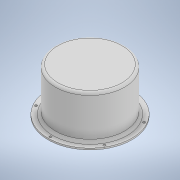
# Autodesk Inventor part: Cover_Joint_1_2
Saved by Autodesk Inventor 2021 (Build 250183000, 183)
## iProperties
Created: 2020-05-10
Part Number: Cover_Joint_1_2
Material: Generic
Document SubType Name: Modeling
Designer: avi41
Density: 1 g/cm^3
Appearance: Default
Mass: 384.639 g
Surface Area: 3507.09 cm^2
Volume: 384.639 cm^3
Author: avi41
Autodesk Inventor part; units mm, degrees
ref_plane "YZ Plane" through (0, 0, 0) normal (1, 0, 0) x (0, 1, 0)
ref_plane "XZ Plane" through (0, 0, 0) normal (0, 1, 0) x (-1, 0, 0)
ref_plane "XY Plane" through (0, 0, 0) normal (0, 0, 1) x (1, 0, 0)
sketch "Sketch1" plane through (0, 0, 0) normal (0, 0, 1) x (1, 0, 0)
  line L0 (-16.3, 0) -> (97.8, 0) construction
  line L1 (0, 60.9) -> (0, -60.9) construction
  line L2 (65.5, -43.5) -> (65.5, 41.5)
  line L3 (81.5, -40.5) -> (81.5, -43.5)
  line L4 (81.5, -43.5) -> (65.5, -43.5)
  line L5 (67.5, -35.5) -> (67.5, 43.5)
  line L6 (81.5, -40.5) -> (72.5, -40.5)
  line L7 (72.5, -40.5) -> (67.5, -35.5)
  line L8 (67.5, 43.5) -> (0, 43.5)
  line L9 (65.5, 41.5) -> (0, 41.5)
  line L10 (0, 43.5) -> (0, 41.5)
  point P0 (0, 0)
  dimension "d5" = 81.5
  dimension "d7" = 9
  dimension "d8" = 5
  dimension "d9" = 45
  dimension "d10" = 16
  dimension "d11" = 3
  dimension "d30" = 2
  dimension "d32" = 2
  dimension "d34" = 87
  constraints: 18 end point, 2 perpendicular, 2 point on line, 1 collinear, 1 horizontal, 1 parallel, 1 vertical, 1 other
  measures "d5" distance between parallel lines of L1 L3
  measures "d7" distance of L3.start L6.end
  measures "d8" horizontal distance of L6.end L5.start
  measures "d9" angle of L4 L7
  measures "d10" distance of L3.end L2.start
  measures "d11" distance between parallel lines of L4 L6
  measures "d30" distance between parallel lines of L9 L8
  measures "d32" distance between parallel lines of L5 L2
  measures "d34" distance between parallel lines of L4 L8
revolve "Revolution1" add sketch "Sketch1" angle 360 about axis through (0, 0, 0) along (0, -1, 0)
sketch "Sketch2" plane through (0, -43.5, 0) normal (0, -1, 0) x (1, 0, 0)
  line L0 (0, 114.1) -> (0, -114.1) construction
  line L1 (-114.1, 0) -> (114.1, 0) construction
  circle A0 centre (0, 0) radius 81.5 construction
  circle A1 centre (0, 0) radius 65.5 construction
  circle A2 centre (0, 0) radius 77 construction
  circle A3 centre (0, 0) radius 72.5 construction
  point P0 (0, 77)
  point P1 (-66.684, 38.5)
  point P2 (-66.684, -38.5)
  point P3 (0, -77)
  point P4 (66.684, -38.5)
  point P5 (66.684, 38.5)
  dimension "d16" = 4.5
  dimension "d20" = 360
  dimension "d29" = 4.5
  constraints: 1 coincident, 1 point on line, 1 vertical alignment, 9 other
hole "Hole1" at (0, -43.5, 77) at (-66.684, -43.5, 38.5) at (-66.684, -43.5, -38.5) at (0, -43.5, -77) at (66.684, -43.5, -38.5) at (66.684, -43.5, 38.5) direction (0, 1, 0) diameter 4.5 depth 13 tip angle 118 clearance for "Flat Head Machine Screw" size "M4" standard "Ansi Metric M Profile"
fillet "Fillet1" radius 5 1 edges at (-67.5, 43.5, 0)
equation "\"d16\" = d29"
body "Solid1"
